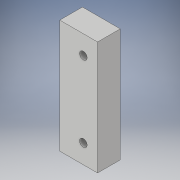
# Autodesk Inventor part: Beefy Spacer
Saved by Autodesk Inventor 2018 (Build 220112000, 112)
## iProperties
Created: 2018-09-30
Part Number: Beefy Spacer
Material: Generic
Document SubType Name: Modeling
Designer: maste
Density: 1 g/cm^3
Appearance: Default
Author: maste
Autodesk Inventor part; units mm, degrees
ref_plane "YZ Plane" through (0, 0, 0) normal (1, 0, 0) x (0, 1, 0)
ref_plane "XZ Plane" through (0, 0, 0) normal (0, 1, 0) x (-1, 0, 0)
ref_plane "XY Plane" through (0, 0, 0) normal (0, 0, 1) x (1, 0, 0)
sketch "Sketch1" plane through (0, 0, 0) normal (0, 0, 1) x (1, 0, 0)
  line L0 (0, 0) -> (25.4, 0)
  line L1 (25.4, 0) -> (25.4, 76.2)
  line L2 (25.4, 76.2) -> (0, 76.2)
  line L3 (0, 76.2) -> (0, 0)
  line L4 (0, 0) -> (6.35, 0)
  line L5 (6.35, 0) -> (6.35, 76.2) construction
  line L6 (6.35, 0) -> (25.4, 0)
  line L7 (15.875, 0) -> (15.875, 76.2) construction
  line L8 (15.875, 0) -> (15.875, 12.7) construction
  line L9 (15.875, 76.2) -> (15.875, 63.5) construction
  circle A0 centre (15.875, 12.7) radius 2.54
  circle A1 centre (15.875, 63.5) radius 2.54
  dimension "d0" = 25.4
  dimension "d1" = 76.2
  dimension "d2" = 6.35
  dimension "d3" = 12.7
  dimension "d4" = 12.7
  dimension "d5" = 5.08
  constraints: 20 end point, 5 point on line, 3 perpendicular, 2 centre point, 2 coincident, 2 parallel, 1 collinear, 1 horizontal, 1 midpoint
  measures "d0" distance of L2.end L1.end
  measures "d1" distance of L1.end L0.end
  measures "d2" distance of L0.start L4.end
  measures "d3" distance of L7.start L8.end
  measures "d4" distance of L7.end L9.end
  measures "d5" diameter of A0
extrude "Extrusion1" add sketch "Sketch1" along normal blind 15.24
body "Solid1"
